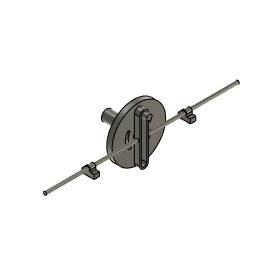
Scotch Yoke mechanism (Autodesk Fusion 360 design; units mm, degrees)
Autodesk Fusion 360 part; units mm, degrees
sketch "Sketch1" plane through (0, 0, 0) normal (1, 0, 0) x (0, 1, 0)
  circle A0 centre (0, 0) radius 50
  circle A1 centre (0, 36) radius 5
  circle A2 centre (0, 0) radius 10
  arc A3 (-17.0596, 10.4389) -> (-14.8427, -13.405) centre (0, 0) ccw
  arc A4 (-21.3244, 13.0487) -> (-18.5534, -16.7562) centre (0, 0) ccw
  arc A5 (-17.0596, 10.4389) -> (-21.3244, 13.0487) centre (-19.192, 11.7438) ccw
  arc A6 (-18.5534, -16.7562) -> (-14.8427, -13.405) centre (-16.6981, -15.0806) ccw
  arc A7 (23.788, -7.6896) -> (19.0304, -6.1517) centre (21.4092, -6.9206) ccw
  arc A8 (-0.5106, -19.9935) -> (-0.6383, -24.9919) centre (-0.5744, -22.4927) ccw
  arc A9 (-0.6383, -24.9919) -> (23.788, -7.6896) centre (0, 0) ccw
  arc A10 (-0.5106, -19.9935) -> (19.0304, -6.1517) centre (0, 0) ccw
  arc A11 (-5.2346, 24.4458) -> (-4.1877, 19.5567) centre (-4.7112, 22.0013) ccw
  arc A12 (17.5702, 9.5545) -> (21.9627, 11.9432) centre (19.7664, 10.7489) ccw
  arc A13 (21.9627, 11.9432) -> (-5.2346, 24.4458) centre (0, 0) ccw
  arc A14 (17.5702, 9.5545) -> (-4.1877, 19.5567) centre (0, 0) ccw
  dimension "d1" = 100
  dimension "d2" = 10
  dimension "d3" = 36
  dimension "d122" = 20
  dimension "d177" = 20
  dimension "d178" = 25
  dimension "d180" = 360
  constraint coincident A0.centre A2.centre
  constraint vertical A0.centre A1.centre
  constraint concentric A2 A3
  constraint tangent A3 A5
  constraint tangent A3 A6
  constraint tangent A4 A5
  constraint tangent A4 A6
  measures "d1" diameter of A0
  measures "d2" diameter of A1
  measures "d3" distance of A0.centre A1.centre
  measures "d122" diameter of A2
  measures "d177" radius of A3
  measures "d178" radius of A4
extrude "Extrude1" add sketch "Sketch1" along normal blind 10 contours A0 | A1 makes body 1
extrude "Extrude2" add sketch "Sketch1" along normal blind 30 contours A1 bodies 1
sketch "Sketch2" plane through (0, 0, 0) normal (1, 0, 0) x (0, 1, 0)
  line L0 (-5, 40) -> (-5, -40)
  arc A0 (-5, -40) -> (5, -40) centre (0, -40) ccw
  line L1 (5, -40) -> (5, 40)
  arc A1 (5, 40) -> (-5, 40) centre (0, 40) ccw
  line L2 (0, 40) -> (0, -40) construction
  line L3 (8, -40) -> (8, 40)
  arc A2 (8, 40) -> (-8, 40) centre (0, 40) ccw
  line L4 (-8, 40) -> (-8, -40)
  arc A3 (-8, -40) -> (8, -40) centre (0, -40) ccw
  dimension "d8" = 5
  dimension "d9" = 80
  dimension "d10" = 3
  constraint tangent L0 A0
  constraint tangent A0 L1
  constraint parallel L0 L1
  constraint tangent L1 A1
  constraint tangent L0 A1
  constraint vertical L2
  constraint coincident origin L2
  constraint midpoint origin L2
  measures "d8" radius of A1
  measures "d9" distance of A1.centre A0.centre
extrude "Extrude3" add sketch "Sketch2" along normal blind 10 separate body makes body 2
move_body "Move1" bodies 2 to x (1, 0, 0) y (0, 1, 0) z (0, 0, 1) at (10, 0, 0)
sketch "Sketch3" plane through (0, 0, 0) normal (1, 0, 0) x (0, 1, 0)
  circle A0 centre (0, 0) radius 10
  dimension "d13" = 20
  constraint coincident A0.centre origin
  measures "d13" diameter of A0
extrude "Extrude4" add sketch "Sketch3" against normal blind 50 separate body makes body 3
copy_body "Body->Comp1" bodies 1 removing the originals makes body 4 in component "Component"
copy_body "Body->Comp2" bodies 2 removing the originals makes body 5 in component "Component'"
copy_body "Body->Comp3" bodies 3 removing the originals makes body 6 in component "Component''"
sketch "Sketch4" plane through (0, 0, 0) normal (0, 1, 0) x (1, 0, 0)
  circle A0 centre (15, 0) radius 3
  line L0 (20, -40) -> (20, 40)
  line L1 (10, -40) -> (20, -40)
  dimension "d40" = 6
  dimension "d41" = 5
  dimension "d42" = 40
  measures "d40" diameter of A0
  measures "d41" distance of A0.centre L0
  measures "d42" distance of A0.centre L1
extrude "Extrude1'" add sketch "Sketch4" along normal blind 180 and the other way blind -5 bodies 5 in component "Component'"
extrude "Extrude2'" add sketch "Sketch4" along normal blind -180 and the other way blind 5 bodies 5 in component "Component'"
sketch "Sketch5" plane through (0, 0, 0) normal (0, 1, 0) x (1, 0, 0)
  circle A0 centre (15.1156, 0.3533) radius 3
  line L0 (19.7797, 0.3533) -> (19.7797, 4.738)
  arc A1 (10.4514, 0.3533) -> (19.7797, 0.3533) centre (15.1156, 0.3533) ccw
  line L1 (15.1156, 0.3533) -> (15.1156, 14.5353) construction
  line L2 (26.4788, 12.6093) -> (3.7524, 12.6093)
  line L3 (3.7524, 12.6093) -> (3.7524, 4.738)
  line L4 (26.4788, 4.738) -> (26.4788, 12.6093)
  line L5 (26.4788, 12.6093) -> (3.7524, 4.738) construction
  line L6 (3.7524, 12.6093) -> (26.4788, 4.738) construction
  line L7 (10.4514, 4.738) -> (10.4514, 0.3533)
  line L8 (3.7524, 4.738) -> (10.4514, 4.738)
  line L9 (19.7797, 4.738) -> (26.4788, 4.738)
  point P0 (15.1156, 8.6736)
  dimension "d51" = 6
  constraint tangent L0 A1
  constraint vertical L1
  constraint coincident A0.centre A1.centre
  constraint horizontal L2
  constraint perpendicular L2 L3
  constraint parallel L2 L8
  constraint parallel L3 L4
  constraint coincident L5 P0
  constraint coincident L6 P0
  constraint coincident L1 P0
  constraint coincident L0.end L8
  constraint collinear L8 L9
  measures "d51" diameter of A0
extrude "Extrude5" add sketch "Sketch5" along normal blind 10 separate body makes body 7
copy_body "Body->Comp4" bodies 7 removing the originals makes body 8 in component "Component'''"
component "Component" placed x (1, 0, 0) y (0, 1, 0) z (0, 0, 1) at (0.1156, 130, 3.6467)
component "Component'" placed x (1, 0, 0) y (0, 1, 0) z (0, 0, 1) at (0.1156, 130, -0.3533)
component "Component''" placed x (1, 0, 0) y (0, 1, 0) z (0, 0, 1) at (0.1156, 130, 3.6467)
component "Component'''" placed x (1, 0, 0) y (0, 1, 0) z (0, 0, 1) at (0, 30, 0)
component "Component'''" placed x (1, 0, 0) y (0, 1, 0) z (0, 0, 1) at (0, 210, 0)
